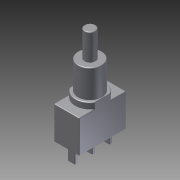
# Autodesk Inventor part: Switch
Saved by Autodesk Inventor 2012 (Build 160160000, 160)
## iProperties
Created: 2016-11-08
Part Number: Switch
Material: Default
Document SubType Name: Modeling
Designer: EGarcia
Density: 1 g/cm^3
Author: EGarcia
Autodesk Inventor part; units mm, degrees
ref_plane "YZ Plane" through (0, 0, 0) normal (1, 0, 0) x (0, 1, 0)
ref_plane "XZ Plane" through (0, 0, 0) normal (0, 1, 0) x (-1, 0, 0)
ref_plane "XY Plane" through (0, 0, 0) normal (0, 0, 1) x (1, 0, 0)
sketch "Boceto1" plane through (0, 0, 0) normal (0, 0, 1) x (1, 0, 0)
  line L0 (0, 0) -> (6.86, 0)
  line L1 (6.86, 0) -> (6.86, 12.7)
  line L2 (6.86, 12.7) -> (0, 12.7)
  line L3 (0, 12.7) -> (0, 0)
  line L4 (3.43, 12.7) -> (3.43, 0)
  circle A0 centre (3.43, 6.35) radius 3.25
  circle A1 centre (3.43, 6.35) radius 1.48
  dimension "d0" = 6.86
  dimension "d1" = 12.7
  dimension "d2" = 6.5
  dimension "d3" = 2.96
  constraints: 10 end point, 3 midpoint, 2 centre point, 2 parallel, 1 coincident, 1 horizontal, 1 perpendicular
  measures "d0" distance of L2.end L1.end
  measures "d1" distance of L1.end L0.end
  measures "d2" diameter of A0
  measures "d3" diameter of A1
extrude "Extrusión1" add sketch "Boceto1" against normal blind 8.9
extrude "Extrusión2" add sketch "Boceto1" along normal blind 16.3 contours A1 L4 | L4 A1
extrude "Extrusión3" add sketch "Boceto1" along normal blind 9.19 contours A0 L4 A1 | L4 A1 A0
sketch "Boceto2" plane through (0, 0, -8.9) normal (0, 0, -1) x (-1, 0, 0)
  line L0 (-2.415, 6.35) -> (-2.415, 6.73)
  line L1 (-2.415, 6.73) -> (-4.445, 6.73)
  line L2 (-4.445, 6.73) -> (-4.445, 5.97)
  line L3 (-4.445, 5.97) -> (-2.415, 5.97)
  line L4 (-2.415, 5.97) -> (-2.415, 6.73)
  line L5 (-3.43, 6.35) -> (-3.43, 1.65)
  line L6 (-2.415, 1.65) -> (-2.415, 2.03)
  line L7 (-2.415, 2.03) -> (-4.445, 2.03)
  line L8 (-4.445, 2.03) -> (-4.445, 1.27)
  line L9 (-4.445, 1.27) -> (-2.415, 1.27)
  line L10 (-2.415, 1.27) -> (-2.415, 2.03)
  line L11 (-2.415, 11.43) -> (-2.415, 10.67)
  line L12 (-4.445, 11.43) -> (-2.415, 11.43)
  line L13 (-4.445, 10.67) -> (-4.445, 11.43)
  line L14 (-2.415, 10.67) -> (-4.445, 10.67)
  line L15 (-2.415, 11.05) -> (-2.415, 10.67)
  point P0 (-3.43, 11.05)
  dimension "d10" = 1.015
  dimension "d11" = 0.38
  dimension "d12" = 2.03
  dimension "d13" = 0.76
  dimension "d14" = 4.7
  dimension "d16" = 0.38
  dimension "d17" = 2.03
  dimension "d18" = 0.76
  constraints: 32 end point, 1 parallel
  measures "d10" distance of L5.start L0.start
  measures "d11" distance of L0.start L0.end
  measures "d12" distance of L0.end L1.end
  measures "d13" distance of L1.end L2.end
  measures "d14" distance of L5.start L5.end
  measures "d16" distance of L6.start L10.end
  measures "d17" distance of L10.end L8.start
  measures "d18" distance of L8.start L9.start
extrude "Extrusión4" add sketch "Boceto2" along normal blind 3.96
sketch "Boceto3" plane through (0, 0, 0) normal (0, 0, 1) x (1, 0, 0)
  circle A0 centre (3.43, 6.35) radius 3.25 projected
  line L0 (6.86, 0) -> (6.86, 12.7) projected
  line L1 (0, 12.7) -> (0, 0) projected
  arc A1 (0, 4.2921) -> (6.86, 4.2921) centre (3.43, 6.35) ccw
  arc A2 (6.86, 8.4079) -> (0, 8.4079) centre (3.43, 6.35) ccw
  line L2 (0, 8.4079) -> (0, 4.2921)
  line L3 (6.86, 8.4079) -> (6.86, 4.2921)
  constraints: 4 end point, 4 point on circle, 4 point on line, 2 centre point, 1 coincident, 1 collinear, 1 parallel
extrude "Extrusión5" add sketch "Boceto3" along normal blind 1.63
fillet "Empalme1" radius 0.2 44 edges at (6.86, 0, -4.45) (0, 0, -4.45) (6.86, 12.7, -4.45) (0, 12.7, -4.45) (3.43, 12.7, -8.9) (6.86, 6.35, -8.9) (0, 6.35, -8.9) (3.43, 0, -8.9) (6.86, 2.146, 0) (6.86, 10.554, 0) (3.43, 12.7, 0) (3.43, 0, 0) (0, 2.146, 0) (0, 10.554, 0) (3.43, 2.35, 1.63) (3.43, 10.35, 1.63) (0.18, 6.35, 9.19) (1.95, 6.35, 16.3) (4.445, 2.03, -10.88) (4.445, 1.27, -10.88) (2.415, 2.03, -10.88) (2.415, 1.27, -10.88) (4.445, 6.73, -10.88) (4.445, 5.97, -10.88) (2.415, 6.73, -10.88) (2.415, 5.97, -10.88) (4.445, 10.67, -10.88) (4.445, 11.43, -10.88) (2.415, 10.67, -10.88) (2.415, 11.43, -10.88) (3.43, 11.43, -12.86) (3.43, 10.67, -12.86) (2.415, 11.05, -12.86) (4.445, 11.05, -12.86) (4.445, 6.35, -12.86) (2.415, 6.35, -12.86) (3.43, 6.73, -12.86) (3.43, 5.97, -12.86) (3.43, 2.03, -12.86) (4.445, 1.65, -12.86) (3.43, 1.27, -12.86) (2.415, 1.65, -12.86) (0, 6.35, 1.63) (6.86, 6.35, 1.63)
